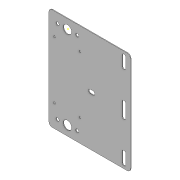
# Autodesk Inventor part: 前方後方板
Saved by Autodesk Inventor 2020.5 (Build 245400000, 400)
## iProperties
Created: 2022-11-26
Part Number: 前方後方板
Material: 一般
Document SubType Name: Modeling
Designer: Administrator
Density: 1 g/cm^3
Appearance: 既定
Author: Administrator
Autodesk Inventor part; units mm, degrees
ref_plane "YZ Plane" through (0, 0, 0) normal (1, 0, 0) x (0, 1, 0)
ref_plane "XZ Plane" through (0, 0, 0) normal (0, 1, 0) x (-1, 0, 0)
ref_plane "XY Plane" through (0, 0, 0) normal (0, 0, 1) x (1, 0, 0)
sketch "スケッチ1" plane through (0, 0, 0) normal (0, 0, 1) x (1, 0, 0)
  circle A0 centre (-15.5, 0) radius 2.5 projected
  circle A1 centre (15.5, 0) radius 2.5 projected
  circle A2 centre (0, 0) radius 11 projected
  line L0 (-15.1987, 13) -> (15.1987, 13) projected
  arc A3 (15.1987, -13) -> (15.1987, 13) centre (0, 0) ccw projected
  line L1 (15.1987, -13) -> (-15.1987, -13) projected
  arc A4 (-15.1987, 13) -> (-15.1987, -13) centre (0, 0) ccw projected
  circle A5 centre (-15.5, -130.182) radius 2.5 projected
  circle A6 centre (15.5, -130.182) radius 2.5 projected
  circle A7 centre (0, -130.182) radius 11 projected
  line L2 (-15.1987, -143.182) -> (15.1987, -143.182) projected
  arc A8 (-15.1987, -117.182) -> (-15.1987, -143.182) centre (0, -130.182) ccw projected
  line L3 (15.1987, -117.182) -> (-15.1987, -117.182) projected
  arc A9 (15.1987, -143.182) -> (15.1987, -117.182) centre (0, -130.182) ccw projected
  circle A10 centre (0, -130.182) radius 5 projected
  circle A11 centre (0, 0) radius 5 projected
  line L4 (-29, -33.3404) -> (-29, 14.9098) projected
  line L5 (99, -145.0893) -> (-29, -145.0893) projected
  line L6 (-29, -63.34) -> (-29, -33.3408)
  line L7 (99, -145.0893) -> (99, 14.9098)
  line L8 (99, 14.9098) -> (297.1795, 14.9098)
  line L9 (297.1795, 14.9098) -> (297.1795, -145.0893)
  line L10 (297.1795, -145.0893) -> (99, -145.0893)
  circle A12 centre (0, -130.1819) radius 55
  circle A13 centre (0, 0.0009) radius 55
  line L11 (297.1795, -145.0893) -> (237.1795, -145.0893)
  line L12 (237.1795, -145.0893) -> (237.1795, 14.9098)
  line L13 (237.1795, 14.9098) -> (297.1795, 14.9098)
  line L14 (297.1795, 14.9098) -> (297.1795, -145.0893)
  line L15 (99, 14.9098) -> (-29, 14.9098) projected
  line L16 (99, 14.9098) -> (99, -145.0893) projected
  line L17 (92, -168.0902) -> (92, 36.9098) projected
  line L18 (86, 36.9098) -> (86, -168.0902) projected
  line L19 (89, 7.9098) -> (89, -7.0902) construction
  line L20 (92, 7.9098) -> (92, -7.0902)
  line L21 (86, -7.0902) -> (86, 7.9098)
  arc A14 (92, 7.9098) -> (86, 7.9098) centre (89, 7.9098) ccw
  arc A15 (86, -7.0902) -> (92, -7.0902) centre (89, -7.0902) ccw
  line L22 (87.3545, -74.7724) -> (87.3545, -54.7724) construction
  line L23 (90.3545, -74.7724) -> (90.3545, -54.7724)
  line L24 (84.3545, -54.7724) -> (84.3545, -74.7724)
  arc A16 (84.3545, -74.7724) -> (90.3545, -74.7724) centre (87.3545, -74.7724) ccw
  arc A17 (90.3545, -54.7724) -> (84.3545, -54.7724) centre (87.3545, -54.7724) ccw
  line L25 (-29, -145.0893) -> (-0.25, -145.0893)
  line L26 (-0.25, -145.0893) -> (-0.25, 14.9098)
  line L27 (-0.25, 14.9098) -> (-29, 14.9098)
  line L28 (-29, 14.9098) -> (-29, -145.0893)
  line L29 (19.75, -105.0893) -> (19.75, -25.0893)
  line L30 (19.75, -25.0893) -> (-20.25, -25.0893)
  line L31 (-20.25, -25.0893) -> (-20.25, -105.0893)
  line L32 (-20.25, -105.0893) -> (19.75, -105.0893)
  line L33 (19.75, -105.0893) -> (-20.25, -25.0893) construction
  line L34 (19.75, -25.0893) -> (-20.25, -105.0893) construction
  line L35 (19.75, -110.0893) -> (19.75, -20.0893)
  line L36 (19.75, -20.0893) -> (-20.25, -20.0893)
  line L37 (-20.25, -20.0893) -> (-20.25, -110.0893)
  line L38 (-20.25, -110.0893) -> (19.75, -110.0893)
  line L39 (19.75, -110.0893) -> (-20.25, -20.0893) construction
  line L40 (19.75, -20.0893) -> (-20.25, -110.0893) construction
  circle A18 centre (19.75, -110.0893) radius 1.5
  circle A19 centre (19.75, -20.0893) radius 1.5
  circle A20 centre (-20.25, -20.0893) radius 1.5
  circle A21 centre (-20.25, -110.0893) radius 1.5
  line L41 (88.9576, -138.0893) -> (88.9576, -123.0893) construction
  line L42 (91.9576, -138.0893) -> (91.9576, -123.0893)
  line L43 (85.9576, -123.0893) -> (85.9576, -138.0893)
  arc A22 (85.9576, -138.0893) -> (91.9576, -138.0893) centre (88.9576, -138.0893) ccw
  arc A23 (91.9576, -123.0893) -> (85.9576, -123.0893) centre (88.9576, -123.0893) ccw
  line L44 (-15.829, -33.3462) -> (-29, -33.3404) projected
  line L45 (-29, -145.0893) -> (-29, -63.34) projected
  line L46 (-29, -63.34) -> (-16.162, -63.34) projected
  arc A24 (-16.162, -63.34) -> (-15.829, -33.3462) centre (-16.25, -48.3403) ccw projected
  line L47 (55.6416, -41.2467) -> (55.6416, -91.2467) projected
  arc A25 (55.6416, -91.2467) -> (80.6416, -91.2467) centre (68.1416, -91.2467) ccw projected
  line L48 (80.6416, -91.2467) -> (80.6416, -41.2467) projected
  arc A26 (80.6416, -41.2467) -> (55.6416, -41.2467) centre (68.1416, -41.2467) ccw projected
  line L49 (86, -55.0898) -> (86, -75.0898) projected
  arc A27 (86, -75.0898) -> (92, -75.0898) centre (89, -75.0898) ccw projected
  line L50 (92, -75.0898) -> (92, -55.0898) projected
  arc A28 (92, -55.0898) -> (86, -55.0898) centre (89, -55.0898) ccw projected
  circle A29 centre (48.7299, -140.0893) radius 1.5 projected
  circle A30 centre (14.75, -81.84) radius 15.8 projected
  circle A31 centre (-15.5, 0.0016) radius 2.5 projected
  circle A32 centre (-15.5, -130.1804) radius 2.5 projected
  arc A33 (86.1416, -121.2458) -> (90.1416, -121.2458) centre (88.1416, -121.2458) ccw projected
  line L51 (90.1416, -121.2458) -> (90.1416, -111.2458) projected
  arc A34 (90.1416, -111.2458) -> (86.1416, -111.2458) centre (88.1416, -111.2458) ccw projected
  line L52 (86.1416, -111.2458) -> (86.1416, -121.2458) projected
  arc A35 (56.1416, -21.2467) -> (60.1416, -21.2467) centre (58.1416, -21.2467) ccw projected
  line L53 (60.1416, -21.2467) -> (60.1416, -11.2467) projected
  arc A36 (60.1416, -11.2467) -> (56.1416, -11.2467) centre (58.1416, -11.2467) ccw projected
  line L54 (56.1416, -11.2467) -> (56.1416, -21.2467) projected
  arc A37 (92, 9.9098) -> (86, 9.9098) centre (89, 9.9098) ccw projected
  line L55 (86, 9.9098) -> (86, -0.0902) projected
  arc A38 (86, -0.0902) -> (92, -0.0902) centre (89, -0.0902) ccw projected
  line L56 (92, -0.0902) -> (92, 9.9098) projected
  arc A39 (56.1416, -121.2458) -> (60.1416, -121.2458) centre (58.1416, -121.2458) ccw projected
  line L57 (60.1416, -121.2458) -> (60.1416, -111.2458) projected
  arc A40 (60.1416, -111.2458) -> (56.1416, -111.2458) centre (58.1416, -111.2458) ccw projected
  line L58 (56.1416, -111.2458) -> (56.1416, -121.2458) projected
  circle A41 centre (68.7415, -140.0893) radius 1.5 projected
  circle A42 centre (0, -130.1803) radius 6.7 projected
  circle A43 centre (15.5, 0.0016) radius 2.5 projected
  circle A44 centre (0, 0.0017) radius 6.7 projected
  circle A45 centre (15.5, -130.1804) radius 2.5 projected
  circle A46 centre (48.73, 9.9098) radius 1.5 projected
  arc A47 (86, -140.0893) -> (92, -140.0893) centre (89, -140.0893) ccw projected
  line L59 (92, -140.0893) -> (92, -130.0893) projected
  arc A48 (92, -130.0893) -> (86, -130.0893) centre (89, -130.0893) ccw projected
  line L60 (86, -130.0893) -> (86, -140.0893) projected
  arc A49 (90.1416, -11.2467) -> (86.1416, -11.2467) centre (88.1416, -11.2467) ccw projected
  line L61 (86.1416, -11.2467) -> (86.1416, -21.2467) projected
  arc A50 (86.1416, -21.2467) -> (90.1416, -21.2467) centre (88.1416, -21.2467) ccw projected
  line L62 (90.1416, -21.2467) -> (90.1416, -11.2467) projected
  line L63 (40.1416, -63.2467) -> (36.1416, -63.2467) projected
  arc A51 (36.1416, -63.2467) -> (36.1416, -69.2467) centre (36.1416, -66.2467) ccw projected
  line L64 (36.1416, -69.2467) -> (40.1416, -69.2467) projected
  arc A52 (40.1416, -69.2467) -> (40.1416, -63.2467) centre (40.1416, -66.2467) ccw projected
  circle A53 centre (68.9885, 9.909) radius 1.5 projected
  circle A54 centre (68.9885, 9.9098) radius 1.5 projected
  line L65 (99, -145.0893) -> (79, -145.0893)
  line L66 (79, -145.0893) -> (79, 14.9098)
  line L67 (79, 14.9098) -> (99, 14.9098)
  line L68 (99, 14.9098) -> (99, -145.0893)
  point P0 (0, 0)
  point P1 (119, 14.909)
  point P2 (89, 0.4098)
  point P3 (92, 7.909)
  point P4 (92, -7.091)
  point P5 (86, -7.094)
  point P6 (86, 7.9142)
  point P7 (87.3545, -64.7724)
  point P8 (86, -7.0941)
  point P9 (86, 7.909)
  point P10 (92, -55.0901)
  point P11 (92, -75.0901)
  point P12 (86, -77.4492)
  point P13 (86, -52.0956)
  point P14 (114.2151, 14.909)
  point P15 (237.2519, 14.9098)
  point P16 (-0.25, -65.0893)
  point P17 (86, -7.0943)
  point P18 (86, -7.091)
  point P19 (88.9576, -130.5893)
  point P20 (86, -138.5921)
  point P21 (86, -122.5866)
  point P22 (112.6121, 14.909)
  point P23 (112.6121, 14.909)
  point P24 (92.6121, -145.0901)
  point P25 (92.6121, 14.909)
  point P26 (-0.25, -145.0901)
  point P27 (92.6121, 14.909)
  point P28 (-0.25, -145.0901)
  point P29 (237.1795, -145.0893)
  point P30 (237.1795, 14.909)
  point P31 (-29, -33.3412)
  point P32 (-29, -63.3408)
  point P33 (-0.25, -145.091)
  point P34 (-29, -33.3422)
  point P35 (-29, -63.3417)
  point P36 (-0.25, -145.091)
  point P37 (-0.25, -145.0908)
  point P38 (-0.25, -145.0908)
  point P39 (-0.25, -145.0905)
  point P40 (-0.25, -145.0905)
  point P41 (-0.25, -145.0902)
  point P42 (-0.25, -145.0902)
  point P43 (-0.25, -145.0899)
  point P44 (-0.25, -145.0899)
  point P45 (-0.25, -145.0896)
  point P46 (-0.25, -145.0896)
  point P47 (-0.25, -145.0893)
  point P48 (-0.25, -145.0893)
  point P49 (-13, -0.0021)
  point P50 (-18, 0.0038)
  point P51 (18, -0.0021)
  point P52 (13, 0.0038)
  point P53 (86, -7.0943)
  point P54 (-13, -130.1782)
  point P55 (-18, -130.1841)
  point P56 (18, -130.1782)
  point P57 (13, -130.1841)
  point P58 (92, -55.0881)
  point P59 (92, -75.0915)
  point P60 (86, -75.0915)
  point P61 (86, -55.0881)
  dimension "d2" = 110
  dimension "d3" = 110
  dimension "d4" = 60
  dimension "d5" = 159.9991
  dimension "d10" = 7
  dimension "d11" = 15
  dimension "d12" = 6
  dimension "d14" = 20
  dimension "d17" = 80
  dimension "d18" = 40
  dimension "d19" = 159.9991
  dimension "d20" = 80
  dimension "d21" = 90
  dimension "d22" = 40
  dimension "d23" = 3
  dimension "d24" = 3
  dimension "d25" = 3
  dimension "d26" = 3
  dimension "d27" = 15
  dimension "d29" = 7
  dimension "d30" = 20
  constraints: 82 end point, 15 parallel, 12 centre point, 12 point on circle, 12 tangent, 7 midpoint, 6 perpendicular, 4 coincident, 4 point on line, 3 vertical, 2 horizontal, 1 other
  measures "d2" diameter of A12
  measures "d3" diameter of A13
  measures "d4" distance of L9.end L11.end
  measures "d5" distance between parallel lines of L13 L11
  measures "d10" distance from line of L15 L19.start
  measures "d11" distance of L19.end L19.start
  measures "d12" diameter of A17
  measures "d14" distance of L22.end L22.start
  measures "d17" distance of L29.start L29.end
  measures "d18" distance of L30.end L29.end
  measures "d19" distance between parallel lines of L15 L5
  measures "d20" distance from line of L5 point (-0.25, -65.089)
  measures "d21" distance of L35.start L35.end
  measures "d22" distance of L36.end L35.end
  measures "d23" diameter of A18
  measures "d24" diameter of A19
  measures "d25" diameter of A20
  measures "d26" diameter of A21
  measures "d27" distance of L41.start L41.end
  measures "d29" distance from line of L11 L41.start
  measures "d30" distance of L66.end L67.end
extrude "押し出し1" add sketch "スケッチ1" along normal blind 1 contours A2 L26 A44 | A2 L26 L0 A3 L1 | L26 A44 A2 | A2 L26 L1 A4 L0 | L26 L15 A13 L29 L35 A19 L36 L1 A3 L0 | L0 A4 L1 L26 L36 A20 L37 L31 L44 L4 L15 | L36 A19 L35 L30 L26 | L26 L30 L37 A20 L36 | L15 L66 A26 L47 A25 L5 A12 A30 L29 A13 | L30 L29 A13 L26 | L26 A13 A24 L44 L31 L30 | L44 L31 A13 L6 | A13 L31 L46 L6 | L15 L18 A17 L24 A16 A23 L43 A22 L5 L66 A25 L48 A26 | L26 A12 L31 L46 A24 A13 | A13 L29 A30 A12 L26 | L44 A24 A13 L31 | L46 L31 A12 L28 | A13 A24 L46 L31 | L15 L17 A37 L18 | L66 A25 L47 A26 | A26 L48 A25 L66 | L26 A30 L32 L31 A12 | A12 A30 L26 | A30 A12 L29 | L29 A12 A30 | A12 L31 L37 A21 L38 L26 L3 A8 L2 L5 L28 | L15 L7 L5 L17 | A37 L17 A14 L18 | A12 L29 A30 L26 | L26 A30 | A12 A30 L29 | L5 L26 L2 A9 L3 L38 A18 L35 L29 A30 A12 | L32 L26 L38 A21 L37 | A30 L29 L32 L26 | L18 A47 L17 L5 | L32 L35 A18 L38 L26 | L26 A7 L3 A9 L2 | L2 A8 L3 L26 A7 | A15 A49 L61 A50 L62 L17 A28 A17 L18 | L18 A22 L42 A48 L17 A47 | L26 A42 A7 | A7 L26 A42 | A17 A28 L18 | L18 A16 L24 A17 | A15 A49 L62 A50 L61 | A22 L43 A23 L18 | A48 L42 A23 L51 A34 L52 A33 L18 A16 A27 L17 | A27 A16 L18 | A33 L52 A34 L51 A23 | A29 | L54 A36 L53 A35 | L58 A40 L57 A39 | A41 | A46 | A53
sketch "スケッチ2" plane through (0, 0, 0) normal (0, 0, -1) x (-1, 0, 0)
  point P0 (0, 0)
fillet "フィレット1" radius 5 4 edges at (-29, -145.0893, 0.5) (-29, 14.9098, 0.5) (99, -145.0893, 0.5) (99, 14.9098, 0.5)
